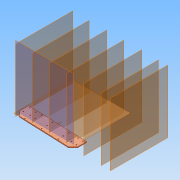
# Autodesk Inventor part: Pancake_Timing Backboard 2_3 Lanes
Saved by Autodesk Inventor 2018.1 (Build 221171000, 171)
## iProperties
Created: 2019-02-22
Part Number: Pancake_Timing Backboard 2_3 Lanes
Material: Wood (Oak)
Document SubType Name: Modeling
Designer: James
Density: 0.76 g/cm^3
Appearance: White Oak - Natural Medium Gloss
Mass: 61.8539 g
Surface Area: 373.467 cm^2
Volume: 81.3867 cm^3
Author: James
Autodesk Inventor part; units mm, degrees
ref_plane "YZ Plane" through (0, 0, 0) normal (1, 0, 0) x (0, 1, 0)
ref_plane "XZ Plane" through (0, 0, 0) normal (0, 1, 0) x (-1, 0, 0)
ref_plane "XY Plane" through (0, 0, 0) normal (0, 0, 1) x (1, 0, 0)
derived "Pancake_Skeleton.ipt"
ref_plane "Ground" through (0, 0, 0) normal (0, 1, 0) x (-1, 0, 0)
ref_plane "Back" through (0, 0, 0) normal (0, 0, 1) x (1, 0, 0)
ref_plane "LHS" through (0, 0, 0) normal (1, 0, 0) x (0, 1, 0)
ref_plane "Lane 1" through (90, 0, 0) normal (1, 0, 0) x (0, 1, 0)
ref_plane "Lane 2" through (185, 0, 0) normal (1, 0, 0) x (0, 1, 0)
ref_plane "Lane 3" through (280, 0, 0) normal (1, 0, 0) x (0, 1, 0)
ref_plane "Lane 4" through (375, 0, 0) normal (1, 0, 0) x (0, 1, 0)
ref_plane "Lane 5" through (470, 0, 0) normal (1, 0, 0) x (0, 1, 0)
ref_plane "RHS" through (520, 0, 0) normal (1, 0, 0) x (0, 1, 0)
sketch "Sketch1" plane through (0, 0, 0) normal (0, 0, 1) x (1, 0, 0)
  line L0 (0, 75.2308) -> (0, -12.5385) projected
  line L1 (0, 12.6923) -> (330, 0)
  line L2 (330, 0) -> (330, 50)
  line L3 (330, 50) -> (0, 62.6923)
  line L4 (0, 62.6923) -> (0, 12.6923)
  line L5 (-66, 0) -> (396, 0) projected
  line L6 (520, 75.2308) -> (520, -12.5385) projected
  dimension "d31" = 50
  dimension "d61" = 2.203
  dimension "d62" = 190
  constraints: 8 end point, 2 parallel, 1 collinear, 1 point on line, 1 vertical
  measures "d31" distance of L1.end L2.end
  measures "d61" angle of L5 L1
  measures "d62" distance between parallel lines of L6 L2
extrude "Extrusion1" add sketch "Sketch1" along normal blind 5 contours L3 L2 L1 L0
sketch "Sketch2" plane through (0, 0, 5) normal (0, 0, 1) x (1, 0, 0)
  line L0 (90, 75.2308) -> (90, -12.5385) projected
  line L1 (330, 50) -> (0, 62.6923) projected
  line L2 (-85, 0) -> (510, 0) projected
  line L3 (185, 79.6154) -> (185, -13.2692) projected
  line L4 (0, 79.6154) -> (0, -13.2692) projected
  line L5 (0, 12.6923) -> (330, 0) projected
  point P0 (0, 0)
  point P1 (50, 50.7692)
  point P2 (50, 20.7692)
  dimension "d4" = 30
  dimension "d29" = 95
  dimension "d30" = 50
  dimension "d33" = 9.9926
  dimension "d34" = 9.9926
  constraints: 1 vertical alignment
  measures "d4" distance of point (50, 20.769) point (50, 50.769)
  measures "d29" distance between parallel lines of L3 L0
  measures "d30" distance from line of point (50, 50.769) L4
  measures "d33" distance from line of L1 point (50, 50.769)
  measures "d34" distance from line of L5 point (50, 20.769)
hole "Hole1" at (50, 50.7692, 5) at (50, 20.7692, 5) direction (0, 0, -1) diameter 4.5 end through all clearance for "Socket Head Cap Screw" size "M4" standard "Ansi Metric M Profile"
pattern_linear "Rectangular Pattern1" count 3 spacing 95 along (0.9992612, -0.0384331, 0) of "Hole1"
sketch "Sketch3" plane through (0, 0, 5) normal (0, 0, 1) x (1, 0, 0)
  line L0 (330, 50) -> (0, 62.6923) projected
  line L1 (-85, 0) -> (510, 0) projected
  line L2 (0, 79.6154) -> (0, -13.2692) projected
  line L3 (0, 12.6923) -> (330, 0) projected
  line L4 (520, 79.6154) -> (520, -13.2692) projected
  line L5 (330, 0) -> (330, 50) projected
  point P0 (0, 0)
  point P1 (12.5, 55.1923)
  point P2 (12.5, 20.1923)
  point P3 (317.5, 42.5)
  point P4 (317.5, 7.5)
  dimension "d20" = 12.5
  dimension "d36" = 35
  dimension "d39" = 35
  dimension "d41" = 7.5
  dimension "d42" = 7.5
  dimension "d63" = 12.5
  constraints: 2 vertical alignment, 1 other
  measures "d20" distance from line of L2 point (12.5, 55.192)
  measures "d36" distance of point (12.5, 20.192) point (12.5, 55.192)
  measures "d39" distance of point (317.5, 7.5) point (317.5, 42.5)
  measures "d41" vertical distance of L0.start point (317.5, 42.5)
  measures "d42" vertical distance of point (12.5, 55.192) L0.end
  measures "d63" distance from line of L5 point (317.5, 42.5)
hole "Hole2" at (12.5, 55.1923, 5) at (12.5, 20.1923, 5) at (317.5, 42.5, 5) at (317.5, 7.5, 5) direction (0, 0, -1) diameter 4.5 end through all clearance for "Socket Head Cap Screw" size "M4" standard "Ansi Metric M Profile"
ref_plane "Work Plane10" through (165, 12.6923, 0) normal (-1, 0, 0) x (0, 0, 1)
sketch "Sketch4" plane through (0, 0, 5) normal (0, 0, 1) x (1, 0, 0)
  line L0 (80, 52.1098) -> (78.6548, 17.1357)
  line L1 (289.8448, 44.0389) -> (288.4997, 9.0647)
  line L2 (330, 50) -> (0, 62.6923) projected
  line L3 (0, 12.6923) -> (330, 0) projected
  line L4 (0, 79.6154) -> (0, -13.2692) projected
  line L5 (520, 79.6154) -> (520, -13.2692) projected
  point P0 (0, 0)
  dimension "d43" = 7.5
  dimension "d44" = 7.5
  dimension "d48" = 35
  dimension "d49" = 80
  dimension "d58" = 35
  dimension "d60" = 210
  constraints: 4 end point, 2 perpendicular, 1 other
  measures "d43" distance from line of L2 L0.start
  measures "d44" distance from line of L2 L1.start
  measures "d48" distance of L0.start L0.end
  measures "d49" distance from line of L0.start L4
  measures "d58" distance of L1.start L1.end
  measures "d60" distance of L1.start L0.start
hole "Hole3" at (80, 52.1098, 5) at (78.6548, 17.1357, 5) at (289.8448, 44.0389, 5) at (288.4997, 9.0647, 5) direction (0, 0, -1) diameter 4.5 end through all clearance for "Flat Head Machine Screw" size "M4" standard "Ansi Metric M Profile"
sketch "Sketch5" plane through (0, 0, 5) normal (0, 0, 1) x (1, 0, 0)
  line L0 (0, 12.6923) -> (330, 0) projected
  line L1 (0, 12.6923) -> (0, -12.3077)
  line L2 (0, -12.3077) -> (330, -25)
  line L3 (330, 0) -> (330, 50) projected
  line L4 (330, -25) -> (330, 0)
  point P0 (0, 0)
  dimension "d64" = 25
  constraints: 6 end point, 2 parallel, 1 vertical
  measures "d64" distance of L2.end L0.end
extrude "Extrusion2" add sketch "Sketch5" against normal up to surface (5 mm away)
sketch "Sketch6" plane through (0, 0, 5) normal (0, 0, 1) x (1, 0, 0)
  circle A0 centre (50, 20.7692) radius 2.25 projected
  point P0 (0, 0)
  point P1 (50, -8.2308)
  dimension "d67" = 29
  constraints: 1 vertical alignment
  measures "d67" distance of point (50, -8.231) A0.centre
hole "Hole4" at (50, -8.2308, 5) direction (0, 0, -1) diameter 4.5 end through all clearance for "Flat Head Machine Screw" size "M4" standard "Ansi Metric M Profile"
pattern_linear "Rectangular Pattern2" count 3 spacing 95 along (0.9992612, -0.0384331, 0) of "Hole4"
chamfer "Chamfer1" distance 25 angle 45 2 edges at (0, -12.3077, 2.5) (330, -25, 2.5)
equation "\"d33\" = d34"
equation "\"d44\" = d43"
equation "\"d58\" = d48"
body "Solid1"
